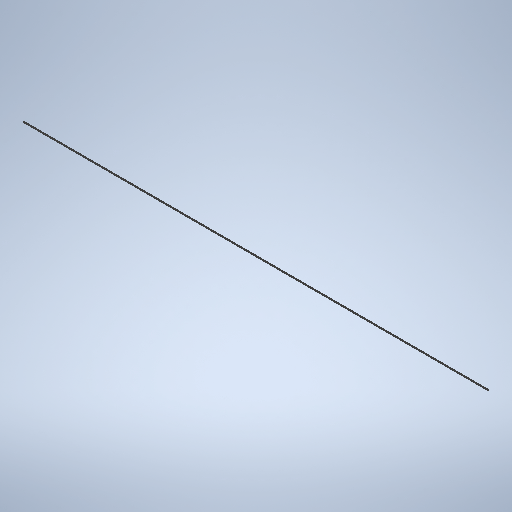
# Autodesk Inventor part: flat 32 gauge nichrome wire
Saved by Autodesk Inventor 2025.1 (Build 291241020, 241B)
## iProperties
Created: 2024-10-29
Part Number: flat 32 gauge nichrome wire
Material: Generic
Document SubType Name: Modeling
Designer: jjk
Density: 1 g/cm^3
Appearance: Default
Author: jjk
Autodesk Inventor part; units mm, degrees
ref_plane "YZ Plane" through (0, 0, 0) normal (1, 0, 0) x (0, 1, 0)
ref_plane "XZ Plane" through (0, 0, 0) normal (0, 1, 0) x (-1, 0, 0)
ref_plane "XY Plane" through (0, 0, 0) normal (0, 0, 1) x (1, 0, 0)
sketch "Sketch1" plane through (0, 0, 0) normal (0, 0, 1) x (1, 0, 0)
  line L0 (0, 0) -> (152.4, 0)
  line L1 (152.4, 0) -> (152.4, 0.2032)
  line L2 (152.4, 0.2032) -> (0, 0.2032)
  line L3 (0, 0.2032) -> (0, 0)
  point P0 (0, 0.1016)
  dimension "d0" = 0.2032
  dimension "d1" = 152.4
  constraints: 8 end point, 2 parallel, 1 horizontal, 1 midpoint, 1 perpendicular
  measures "d0" distance between parallel lines of L0 L2
  measures "d1" distance from line of point (0, 0.102) L1
extrude "Extrusion1" add sketch "Sketch1" along normal blind 0.2032
body "Solid1"
